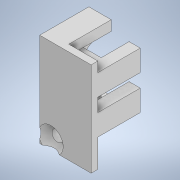
# Autodesk Inventor part: encoderholder
Saved by Autodesk Inventor 2022 (Build 260153000, 153)
## iProperties
Created: 2021-01-11
Part Number: encoderholder
Material: Generic
Document SubType Name: Modeling
Designer: papa
Density: 1 g/cm^3
Appearance: Default
Author: papa
Autodesk Inventor part; units mm, degrees
ref_plane "YZ Plane" through (0, 0, 0) normal (1, 0, 0) x (0, 1, 0)
ref_plane "XZ Plane" through (0, 0, 0) normal (0, 1, 0) x (-1, 0, 0)
ref_plane "XY Plane" through (0, 0, 0) normal (0, 0, 1) x (1, 0, 0)
sketch "Sketch1" plane through (0, 0, 0) normal (0, 0, 1) x (1, 0, 0)
  line L0 (73, 108.5) -> (85, 108.5)
  line L1 (85, 108.5) -> (85, 130.5)
  line L2 (85, 130.5) -> (73, 130.5)
  line L3 (73, 130.5) -> (73, 108.5)
  line L4 (82, 115.25) -> (82, 120)
  line L5 (85, 115.25) -> (78, 115.25)
  line L6 (82, 120) -> (85, 120)
  line L7 (85, 120) -> (85, 115.25)
  line L8 (85, 115.25) -> (82, 115.25)
  line L9 (82, 115.25) -> (82, 120)
  line L10 (78, 127.75) -> (85, 127.75)
  line L11 (82, 127.75) -> (85, 127.75)
  line L12 (85, 127.75) -> (85, 123)
  line L13 (85, 123) -> (82, 123)
  line L14 (82, 123) -> (82, 127.75)
  line L15 (78, 115.25) -> (78, 108.5)
  line L16 (73, 130.5) -> (78, 130.5)
  line L17 (78, 108.5) -> (73, 108.5)
  line L18 (73, 108.5) -> (73, 130.5)
  line L19 (73, 130.5) -> (78, 130.5)
  line L20 (75, 125) -> (75, 127.75)
  line L21 (78, 115.25) -> (75, 115.25)
  line L22 (75, 115.25) -> (75, 127.75)
  line L23 (75, 127.75) -> (78, 127.75)
  line L24 (78, 130.5) -> (78, 127.75)
  line L25 (78, 115.25) -> (78, 108.5)
  circle A0 centre (75.5, 111) radius 1.25
  dimension "d0" = 6.75
  dimension "d1" = 2.75
  dimension "d2" = 2
  dimension "d3" = 3
  dimension "d5" = 3
  dimension "d6" = 4
  dimension "d7" = 3
  dimension "d8" = 2.5
  dimension "d9" = 2.5
  dimension "d10" = 2.5
  constraints: 52 end point, 10 parallel, 5 horizontal, 5 perpendicular, 4 point on line, 3 collinear, 1 centre point
  measures "d0" distance between parallel lines of L0 L21
  measures "d1" distance between parallel lines of L2 L23
  measures "d2" distance between parallel lines of L3 L22
  measures "d3" distance between parallel lines of L12 L14
  measures "d5" distance from line of L20.start L24
  measures "d6" distance between parallel lines of L24 L14
  measures "d7" distance between parallel lines of L6 L13
  measures "d8" distance from line of L0 A0.centre
  measures "d9" distance from line of L18 A0.centre
  measures "d10" diameter of A0
extrude "Extrusion1" add sketch "Sketch1" against normal blind 9.5 contours L3 L2 L24 L23 L20 L22 L21 L15 L0 | L5 L4 L6 L1 | L1 L13 L14 L10
extrude "Extrusion2" add sketch "Sketch1" along normal blind 1.5
sketch "Sketch2" plane through (75, 115.25, -9.5) normal (1, 0, 0) x (0, 0, -1)
  line L0 (0, 12.5) -> (0, 0) projected
  circle A0 centre (0, 6.25) radius 3.5
  point P0 (0, 2.75)
  point P1 (0, 9.75)
  dimension "d15" = 7
  constraints: 1 centre point, 1 midpoint
  measures "d15" diameter of A0
extrude "Extrusion3" cut sketch "Sketch2" against normal through all contours L0 A0 picked at (-2.1437, 6.9232)
sketch "Sketch3" plane through (0, 0, 0) normal (0, 0, -1) x (-1, 0, 0)
  line L0 (-75, 115.25) -> (-75, 127.75) projected
  line L1 (-82, 115.25) -> (-82, 120) projected
  line L2 (-75, 127.75) -> (-82, 127.75)
  line L3 (-82, 127.75) -> (-82, 115.25)
  line L4 (-82, 115.25) -> (-75, 115.25)
  line L5 (-75, 115.25) -> (-75, 127.75)
  point P0 (0, 0)
  constraints: 8 end point, 2 parallel, 1 horizontal, 1 perpendicular
extrude "Extrusion4" add sketch "Sketch3" along normal blind 3.25
thicken "Thicken2" operation add thickness 0.5 both sides no extend neighbours yes toward (0, -1, 0) faces at (74.6667, 130.5, -2.6667) (85, 116.8333, -3.1667) (74.6667, 108.5, -2.6667)
chamfer "Chamfer1" distance 1.5 angle 45 1 edges at (74.25, 111, 1.5)
body "Solid1"
